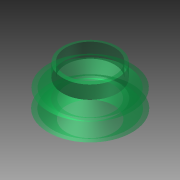
# Autodesk Inventor part: Small Suction Cup Part 1 1764
Saved by Autodesk Inventor 2011 (Build 150239000, 239)
## iProperties
Created: 2011-01-15
Part Number: Small Suction Cup Part 1 1764
Document SubType Name: Modeling
Designer: dfranz
Density: 1 g/cm^3
Author: dfranz
Autodesk Inventor part; units mm, degrees
ref_plane "YZ Plane" through (0, 0, 0) normal (1, 0, 0) x (0, 1, 0)
ref_plane "XZ Plane" through (0, 0, 0) normal (0, 1, 0) x (-1, 0, 0)
ref_plane "XY Plane" through (0, 0, 0) normal (0, 0, 1) x (1, 0, 0)
sketch "Sketch1" plane through (0, 0, 0) normal (0, 0, 1) x (1, 0, 0)
  line L0 (-45.1128, 14.1503) -> (-50.5079, 10.8014)
  line L1 (-50.5079, 10.8014) -> (-45.2136, 7.2953)
  line L2 (-45.2136, 7.2953) -> (-50.6087, 3.9464)
  line L3 (-50.6087, 3.9464) -> (-45.3144, 0.4403)
  line L4 (-45.1128, 14.1503) -> (-45.1128, 19.2303)
  line L5 (-43.8697, 19.4903) -> (-45.1128, 19.2303)
  line L6 (-34.6329, 29.115) -> (-34.6329, -7.5025)
  line L7 (-43.8697, 13.8605) -> (-48.8373, 10.7769)
  line L8 (-48.8373, 10.7769) -> (-43.543, 7.2708)
  line L9 (-43.543, 7.2708) -> (-48.9149, 3.9362)
  line L10 (-43.8697, 19.4903) -> (-43.8697, 13.8605)
  line L11 (-48.9149, 3.9362) -> (-43.6359, 0.4403)
  line L12 (-43.6359, 0.4403) -> (-45.3144, 0.4403)
  point P0 (0, 0)
  dimension "d0" = 6.35
  dimension "d1" = 6.35
  dimension "d2" = 5.08
  dimension "d3" = 1.27
  dimension "d4" = 15.875
  dimension "d6" = 6.35
  dimension "d10" = 1.6784
  dimension "d11" = 19.05
  constraints: 26 end point, 5 parallel, 2 equal length, 2 vertical, 1 perpendicular, 2 other
  measures "d0" distance of L0.start L0.end
  measures "d1" distance of L0.end L1.end
  measures "d2" distance of L0.start L4.end
  measures "d3" distance of L5.start L4.end
  measures "d4" distance from line of L0.end L6
  measures "d6" distance of L1.end L2.end
  measures "d10" distance of L11.end L3.end
  measures "d11" distance from line of L12 L5.start
revolve "Revolution1" add sketch "Sketch1" angle 360 about axis through (-34.6329, 29.115, 0) along (0, -1, 0)
body "Solid1"
